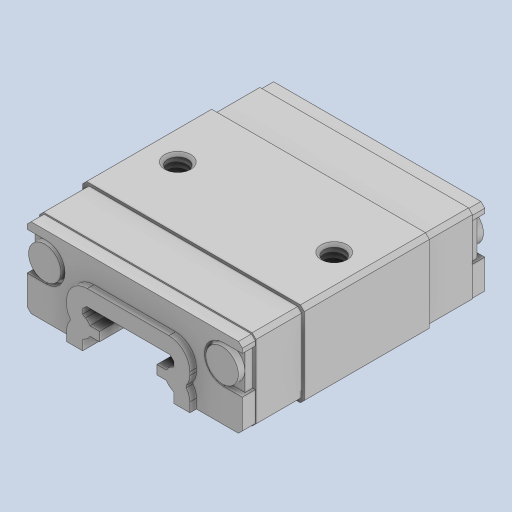
# Autodesk Inventor part: SEBSZ8_b
Saved by Autodesk Inventor 2023 (Build 270158000, 158)
## iProperties
Category: PARTsolutions
Company: MISUMI
Created: 2024-12-13
Part Number: SEBSZ8_b
Material: Generic
Catalog Web Link: www.cadenas.de
Description: SEBSZ, SE2BSZ, SSEBSZ, SSEBSZ-MX, SSE2BSZ, SSE2BSLZ-MX, SEBSLZ, SE2BSLZ, SSEBSLZ, SSEBSZ-MX, SSE2BSLZ, SSE2BSLZ-MX_block-Miniature Linear Guides - Short Block, Standard Preload
Vendor: MISUMI
Document SubType Name: Modeling
Designer: psAdmin
Manufacturer: MISUMI
Mass: 1.60852 g
Surface Area: 13.4851 cm^2
Volume: 1.60852 cm^3
Density: 1 g/cm^3
Appearance: PSOLRGB-175-175-175
PSOL_IDENT_0: {$CADENAS_DATA/23d-libs/misumi/metric/06_linear_guides/sebsz_series/sebsz_block.prj},277 {VTYP=3D},{
PSOL_IDENT_1: NB=SEBSZ8_b},{LINA=SEBSZ8},{NN=SEBSZ, SE2BSZ, SSEBSZ, SSEBSZ-MX, SSE2BSZ, SSE2BSLZ-MX, SEBSLZ, SE2BS
PSOL_IDENT_2: LZ, SSEBSLZ, SSEBSZ-MX, SSE2BSLZ, SSE2BSLZ-MX_block},{DATE=01.06.2021 05:33:07},{GEOMDATE=28.09.2020
PSOL_IDENT_3: 00:26:00},{VERSION=},{LINEID=90},{WBVAR=MAT,ST,MX},{WBNUMERIC=}  {NB=SEBSZ8_b},{LINA=SEBSZ8},{KT=DU
PSOL_IDENT_4: MMY},{PN=SEBSZ8},{TYPE=SEBSZ},{H=8},{MAT=S},{ST=S},{ST1='S', 'w/o Surface Treatment','R','Low Temper
PSOL_IDENT_5: ature Black Chrome Plating'},{MX=},{MXALG= '','w/o MX(Lubrication unit)' },{HARD=56HRC~},{STPN=},{W=
PSOL_IDENT_6: 17},{L1=19.6},{B=12},{SLL=M2x2.5},{S=2},{LL=2.5},{L2=9.6},{K=6.5},{CBB=0.3},{W1=7},{W2=5.0},{H1=4.7}
PSOL_IDENT_7: ,{CAA=0.3},{F=15},{G=5.0},{CA1=0.3},{CA2=0.3},{VA1=1.5},{HA1=1.3},{WA1=1.6677},{WA2=0.7},{RA1=1.75},
PSOL_IDENT_8: {HA2=7.4140},{POIA1=0.1140},{BHA1=13.6},{BHA2=16.5},{BHA3=16.6},{BHA5=9.7445},{BHA6=16.1},{BHA7=0.0}
PSOL_IDENT_9: ,{BHA8=0.0},{BVA1=2.40},{BVA3=0.20},{BVA4=0.30},{BVA5=6.10},{BVA6=6.20},{BCA1=0.3},{BCA2H=0.00},{BCA
PSOL_IDENT_10: 2V=0.00},{BRA1=1.45},{BRA2=1.25},{BDA1=25.00},{BHB1=9.4600},{BHB2=8.9100},{BVB1=4.3300},{BVB2=1.7485
PSOL_IDENT_11: },{BRB1=1.6},{BRB2=1.3000},{BRB3=0.0},{BHC1=3.50},{BHC2=1.0},{BHC3=0.5},{BHC4=0.4},{BHC5=0.5},{MD=5.
PSOL_IDENT_12: 5}
NB: SEBSZ8_b
NN: SEBSZ, SE2BSZ, SSEBSZ, SSEBSZ-MX, SSE2BSZ, SSE2BSLZ-MX, SEBSLZ, SE2BSLZ, SSEBSLZ, SSEBSZ-MX, SSE2BSLZ, SSE2BSLZ-MX_block
NT: Miniature Linear Guides - Short Block, Standard Preload
NBSYN: $PN._b
LINA: SEBSZ8
CATALOG: Misumi
PN: SEBSZ8
H: 8
MAT: Stainless Steel
ST: w/o Surface Treatment
MX: w/o MX(Lubrication unit)
W: 17
L1: 19.6
B: 12
SLL: M2x2.5
S: 2
LL: 2.5
L2: 9.6
K: 6.5
CBB: 0.3
W1: 7
W2: 5
H1: 4.7
CAA: 0.3
F: 15
G: 5
CA1: 0.3
CA2: 0.3
VA1: 1.5
HA1: 1.3
WA1: 1.6677
WA2: 0.7
RA1: 1.75
HA2: 7.414
POIA1: 0.114
BHA1: 13.6
BHA2: 16.5
BHA3: 16.6
BHA5: 9.7445
BHA6: 16.1
BHA7: 0
BHA8: 0
BVA1: 2.4
BVA3: 0.2
BVA4: 0.3
BVA5: 6.1
BVA6: 6.2
BCA1: 0.3
BCA2H: 0
BCA2V: 0
BRA1: 1.45
BRA2: 1.25
BDA1: 25
BHB1: 9.46
BHB2: 8.91
BVB1: 4.33
BVB2: 1.7485
BRB1: 1.6
BRB2: 1.3
BRB3: 0
BHC1: 3.5
BHC2: 1
BHC3: 0.5
BHC4: 0.4
BHC5: 0.5
MD: 5.5
SUPPLIER: MISUMI
ARTICLENO: SEBSZ8_b
BOMINFO: SEBSZ8
CREATOR: CADENAS GmbH
Title: SEBSZ8
Author: Cadenas PARTsolutions
Comments: Miniature Linear Guides - Short Block, Standard Preload
Autodesk Inventor part; units mm, degrees
ref_plane "YZ Plane" through (0, 0, 0) normal (1, 0, 0) x (0, 1, 0)
ref_plane "XZ Plane" through (0, 0, 0) normal (0, 1, 0) x (-1, 0, 0)
ref_plane "XY Plane" through (0, 0, 0) normal (0, 0, 1) x (1, 0, 0)
sketch "Sketch_1" plane through (0, 0, 0) normal (0, 0, 1) x (1, 0, 0)
  line L0 (-8.5, 1.8) -> (-8.2, 1.5)
  line L1 (-8.2, 1.5) -> (-4.8723, 1.5)
  line L2 (-4.8723, 1.5) -> (-4.6578, 1.6)
  line L3 (-4.6578, 1.6) -> (4.6578, 1.6)
  line L4 (4.6578, 1.6) -> (4.8723, 1.5)
  line L5 (4.8723, 1.5) -> (8.2, 1.5)
  line L6 (8.2, 1.5) -> (8.5, 1.8)
  line L7 (8.5, 1.8) -> (8.5, 7.7)
  line L8 (8.5, 7.7) -> (8.2, 8)
  line L9 (8.2, 8) -> (-8.2, 8)
  line L10 (-8.2, 8) -> (-8.5, 7.7)
  line L11 (-8.5, 7.7) -> (-8.5, 1.8)
  constraints: 24 end point
extrude "Extrusion1" add sketch "Sketch_1" along normal mid plane 9.6
sketch "Sketch_3" plane through (0, 0, 4.8) normal (0, 0, 1) x (1, 0, 0)
  line L0 (-8.3, 7.5) -> (-8.3, 1.9)
  line L1 (-8.3, 1.9) -> (-8, 1.6)
  line L2 (-8, 1.6) -> (8, 1.6)
  line L3 (8, 1.6) -> (8.3, 1.9)
  line L4 (8.3, 1.9) -> (8.3, 7.5)
  line L5 (8.3, 7.5) -> (8, 7.8)
  line L6 (8, 7.8) -> (-8, 7.8)
  line L7 (-8, 7.8) -> (-8.3, 7.5)
  constraints: 16 end point
extrude "Extrusion2" add sketch "Sketch_3" along normal blind 5
sketch "Sketch_4" plane through (0, 0, -4.8) normal (0, 0, 1) x (1, 0, 0)
  line L0 (-8.3, 7.5) -> (-8.3, 1.9)
  line L1 (-8.3, 1.9) -> (-8, 1.6)
  line L2 (-8, 1.6) -> (8, 1.6)
  line L3 (8, 1.6) -> (8.3, 1.9)
  line L4 (8.3, 1.9) -> (8.3, 7.5)
  line L5 (8.3, 7.5) -> (8, 7.8)
  line L6 (8, 7.8) -> (-8, 7.8)
  line L7 (-8, 7.8) -> (-8.3, 7.5)
  constraints: 16 end point
extrude "Extrusion3" add sketch "Sketch_4" against normal blind 5
sketch "Sketch_8" plane through (0, 0, 9.8) normal (0, 0, 1) x (1, 0, 0)
  line L0 (-17, 12) -> (-17, 0)
  line L1 (-17, 0) -> (17, 0)
  line L2 (17, 0) -> (17, 12)
  line L3 (17, 12) -> (-17, 12)
  line L4 (-8.25, 7.05) -> (-6.8, 7.05)
  arc A0 (-6.8, 4.15) -> (-6.8, 7.05) centre (-6.8, 5.6) ccw
  line L5 (-6.8, 4.15) -> (-8.25, 4.15)
  line L6 (-8.25, 4.15) -> (-8.25, 1.9)
  line L7 (-8.25, 1.9) -> (-7.95, 1.6)
  line L8 (-7.95, 1.6) -> (7.95, 1.6)
  line L9 (7.95, 1.6) -> (8.25, 1.9)
  line L10 (8.25, 1.9) -> (8.25, 4.15)
  line L11 (8.25, 4.15) -> (6.8, 4.15)
  arc A1 (6.8, 7.05) -> (6.8, 4.15) centre (6.8, 5.6) ccw
  line L12 (6.8, 7.05) -> (8.25, 7.05)
  line L13 (8.25, 7.05) -> (8.25, 7.4)
  line L14 (8.25, 7.4) -> (7.95, 7.7)
  line L15 (7.95, 7.7) -> (-7.95, 7.7)
  line L16 (-7.95, 7.7) -> (-8.25, 7.4)
  line L17 (-8.25, 7.4) -> (-8.25, 7.05)
  constraints: 36 end point, 4 point on circle, 2 centre point
extrude "Extrusion4" cut sketch "Sketch_8" against normal blind 1.5
sketch "Sketch_6" plane through (0, 0, 9.8) normal (0, 0, 1) x (1, 0, 0)
  line L0 (-17, 11.2) -> (-17, 1.6)
  line L1 (-17, 1.6) -> (-4.73, 1.6)
  line L2 (-4.73, 1.6) -> (-4.73, 2.3258)
  arc A0 (-4.455, 3.1254) -> (-4.73, 2.3258) centre (-3.43, 2.3257) ccw
  line L3 (-4.455, 3.1254) -> (-4.455, 3.2746)
  arc A1 (-4.73, 4.0743) -> (-4.455, 3.2746) centre (-3.43, 4.0743) ccw
  line L4 (-4.73, 4.0743) -> (-4.73, 4.33)
  arc A2 (-3.13, 5.93) -> (-4.73, 4.33) centre (-3.13, 4.33) ccw
  line L5 (-3.13, 5.93) -> (3.13, 5.93)
  arc A3 (4.73, 4.33) -> (3.13, 5.93) centre (3.13, 4.33) ccw
  line L6 (4.73, 4.33) -> (4.73, 4.0743)
  arc A4 (4.455, 3.2746) -> (4.73, 4.0743) centre (3.43, 4.0743) ccw
  line L7 (4.455, 3.2746) -> (4.455, 3.1254)
  arc A5 (4.73, 2.3258) -> (4.455, 3.1254) centre (3.43, 2.3257) ccw
  line L8 (4.73, 2.3258) -> (4.73, 1.6)
  line L9 (4.73, 1.6) -> (17, 1.6)
  line L10 (17, 1.6) -> (17, 11.2)
  line L11 (17, 11.2) -> (-17, 11.2)
  constraints: 24 end point, 12 point on circle, 6 centre point
extrude "Extrusion5" cut sketch "Sketch_6" against normal blind 0.5
sketch "Sketch_7" plane through (0, 0, -9.8) normal (0, 0, 1) x (1, 0, 0)
  line L0 (-17, 12) -> (-17, 0)
  line L1 (-17, 0) -> (17, 0)
  line L2 (17, 0) -> (17, 12)
  line L3 (17, 12) -> (-17, 12)
  line L4 (-8.25, 7.05) -> (-6.8, 7.05)
  arc A0 (-6.8, 4.15) -> (-6.8, 7.05) centre (-6.8, 5.6) ccw
  line L5 (-6.8, 4.15) -> (-8.25, 4.15)
  line L6 (-8.25, 4.15) -> (-8.25, 1.9)
  line L7 (-8.25, 1.9) -> (-7.95, 1.6)
  line L8 (-7.95, 1.6) -> (7.95, 1.6)
  line L9 (7.95, 1.6) -> (8.25, 1.9)
  line L10 (8.25, 1.9) -> (8.25, 4.15)
  line L11 (8.25, 4.15) -> (6.8, 4.15)
  arc A1 (6.8, 7.05) -> (6.8, 4.15) centre (6.8, 5.6) ccw
  line L12 (6.8, 7.05) -> (8.25, 7.05)
  line L13 (8.25, 7.05) -> (8.25, 7.4)
  line L14 (8.25, 7.4) -> (7.95, 7.7)
  line L15 (7.95, 7.7) -> (-7.95, 7.7)
  line L16 (-7.95, 7.7) -> (-8.25, 7.4)
  line L17 (-8.25, 7.4) -> (-8.25, 7.05)
  constraints: 36 end point, 4 point on circle, 2 centre point
extrude "Extrusion6" cut sketch "Sketch_7" along normal blind 1.5
sketch "Sketch_12" plane through (0, 0, -9.8) normal (0, 0, 1) x (1, 0, 0)
  line L0 (-17, 11.2) -> (-17, 1.6)
  line L1 (-17, 1.6) -> (-4.73, 1.6)
  line L2 (-4.73, 1.6) -> (-4.73, 2.3258)
  arc A0 (-4.455, 3.1254) -> (-4.73, 2.3258) centre (-3.43, 2.3257) ccw
  line L3 (-4.455, 3.1254) -> (-4.455, 3.2746)
  arc A1 (-4.73, 4.0743) -> (-4.455, 3.2746) centre (-3.43, 4.0743) ccw
  line L4 (-4.73, 4.0743) -> (-4.73, 4.33)
  arc A2 (-3.13, 5.93) -> (-4.73, 4.33) centre (-3.13, 4.33) ccw
  line L5 (-3.13, 5.93) -> (3.13, 5.93)
  arc A3 (4.73, 4.33) -> (3.13, 5.93) centre (3.13, 4.33) ccw
  line L6 (4.73, 4.33) -> (4.73, 4.0743)
  arc A4 (4.455, 3.2746) -> (4.73, 4.0743) centre (3.43, 4.0743) ccw
  line L7 (4.455, 3.2746) -> (4.455, 3.1254)
  arc A5 (4.73, 2.3258) -> (4.455, 3.1254) centre (3.43, 2.3257) ccw
  line L8 (4.73, 2.3258) -> (4.73, 1.6)
  line L9 (4.73, 1.6) -> (17, 1.6)
  line L10 (17, 1.6) -> (17, 11.2)
  line L11 (17, 11.2) -> (-17, 11.2)
  constraints: 24 end point, 12 point on circle, 6 centre point
extrude "Extrusion7" cut sketch "Sketch_12" along normal blind 0.5
sketch "Sketch_25" plane through (0, 0, 8.3) normal (0, 0, 1) x (1, 0, 0)
  line L0 (-8.05, 7.05) -> (-8.05, 4.15)
  line L1 (-8.05, 4.15) -> (-6.8, 4.15)
  arc A0 (-6.8, 4.15) -> (-6.8, 7.05) centre (-6.8, 5.6) ccw
  line L2 (-6.8, 7.05) -> (-8.05, 7.05)
  constraints: 6 end point, 2 point on circle, 1 centre point
extrude "Extrusion8" add sketch "Sketch_25" along normal blind 0.6
sketch "Sketch_5" plane through (0, 0, 8.3) normal (0, 0, 1) x (1, 0, 0)
  arc A0 (6.8, 7.05) -> (6.8, 4.15) centre (6.8, 5.6) ccw
  line L0 (6.8, 4.15) -> (8.05, 4.15)
  line L1 (8.05, 4.15) -> (8.05, 7.05)
  line L2 (8.05, 7.05) -> (6.8, 7.05)
  constraints: 6 end point, 2 point on circle, 1 centre point
extrude "Extrusion9" add sketch "Sketch_5" along normal blind 0.6
sketch "Sketch_9" plane through (0, 0, -8.3) normal (0, 0, 1) x (1, 0, 0)
  line L0 (-8.05, 7.05) -> (-8.05, 4.15)
  line L1 (-8.05, 4.15) -> (-6.8, 4.15)
  arc A0 (-6.8, 4.15) -> (-6.8, 7.05) centre (-6.8, 5.6) ccw
  line L2 (-6.8, 7.05) -> (-8.05, 7.05)
  constraints: 6 end point, 2 point on circle, 1 centre point
extrude "Extrusion10" add sketch "Sketch_9" against normal blind 0.6
sketch "Sketch_26" plane through (0, 0, -8.3) normal (0, 0, 1) x (1, 0, 0)
  arc A0 (6.8, 7.05) -> (6.8, 4.15) centre (6.8, 5.6) ccw
  line L0 (6.8, 4.15) -> (8.05, 4.15)
  line L1 (8.05, 4.15) -> (8.05, 7.05)
  line L2 (8.05, 7.05) -> (6.8, 7.05)
  constraints: 6 end point, 2 point on circle, 1 centre point
extrude "Extrusion11" add sketch "Sketch_26" against normal blind 0.6
sketch "Sketch_18" plane through (-6.8, 0, 0) normal (1, 0, 0) x (0, 0, -1)
  line L0 (-8.9, 5.6) -> (-9.4, 5.6)
  line L1 (-9.4, 5.6) -> (-9.4, 6.85)
  line L2 (-9.4, 6.85) -> (-8.9, 6.85)
  line L3 (-8.9, 6.85) -> (-8.9, 5.6)
  line L4 (-8.9, 5.6) -> (-9.4, 5.6)
  constraints: 10 end point
revolve "Revolution1" add sketch "Sketch_18" angle 360 about axis through (-6.8, 5.6, 8.9) along (0, 0, -1)
sketch "Sketch_19" plane through (-6.8, 0, 0) normal (1, 0, 0) x (0, 0, -1)
  line L0 (9.4, 5.6) -> (8.9, 5.6)
  line L1 (8.9, 5.6) -> (8.9, 6.85)
  line L2 (8.9, 6.85) -> (9.4, 6.85)
  line L3 (9.4, 6.85) -> (9.4, 5.6)
  line L4 (9.4, 5.6) -> (8.9, 5.6)
  constraints: 10 end point
revolve "Revolution2" add sketch "Sketch_19" angle 360 about axis through (-6.8, 5.6, -9.4) along (0, 0, -1)
sketch "Sketch_20" plane through (6.8, 0, 0) normal (1, 0, 0) x (0, 0, -1)
  line L0 (-8.9, 5.6) -> (-9.4, 5.6)
  line L1 (-9.4, 5.6) -> (-9.4, 6.85)
  line L2 (-9.4, 6.85) -> (-8.9, 6.85)
  line L3 (-8.9, 6.85) -> (-8.9, 5.6)
  line L4 (-8.9, 5.6) -> (-9.4, 5.6)
  constraints: 10 end point
revolve "Revolution3" add sketch "Sketch_20" angle 360 about axis through (6.8, 5.6, 8.9) along (0, 0, -1)
sketch "Sketch_21" plane through (6.8, 0, 0) normal (1, 0, 0) x (0, 0, -1)
  line L0 (9.4, 5.6) -> (8.9, 5.6)
  line L1 (8.9, 5.6) -> (8.9, 6.85)
  line L2 (8.9, 6.85) -> (9.4, 6.85)
  line L3 (9.4, 6.85) -> (9.4, 5.6)
  line L4 (9.4, 5.6) -> (8.9, 5.6)
  constraints: 10 end point
revolve "Revolution4" add sketch "Sketch_21" angle 360 about axis through (6.8, 5.6, -9.4) along (0, 0, -1)
sketch "Sketch_17" plane through (0, 0, 0) normal (0, 0, 1) x (1, 0, 0)
  line L0 (-3.5, 4.4) -> (-3.5, 4.0339)
  line L1 (-3.5, 4.0339) -> (-3.2695, 3.9008)
  arc A0 (-2.9324, 3.55) -> (-3.2695, 3.9008) centre (-3.707, 3.143) ccw
  line L2 (-2.9324, 3.55) -> (-2.2, 3.55)
  line L3 (-2.2, 3.55) -> (-2.2, 2.85)
  line L4 (-2.2, 2.85) -> (-2.9324, 2.85)
  arc A1 (-3.2695, 2.4992) -> (-2.9324, 2.85) centre (-3.707, 3.257) ccw
  line L5 (-3.2695, 2.4992) -> (-3.5, 2.3662)
  line L6 (-3.5, 2.3662) -> (-3.5, 0.3)
  line L7 (-3.5, 0.3) -> (-3.2, 0)
  line L8 (-3.2, 0) -> (3.2, 0)
  line L9 (3.2, 0) -> (3.5, 0.3)
  line L10 (3.5, 0.3) -> (3.5, 2.3662)
  line L11 (3.5, 2.3662) -> (3.2695, 2.4992)
  arc A2 (2.9324, 2.85) -> (3.2695, 2.4992) centre (3.707, 3.257) ccw
  line L12 (2.9324, 2.85) -> (2.2, 2.85)
  line L13 (2.2, 2.85) -> (2.2, 3.55)
  line L14 (2.2, 3.55) -> (2.9324, 3.55)
  arc A3 (3.2695, 3.9008) -> (2.9324, 3.55) centre (3.707, 3.143) ccw
  line L15 (3.2695, 3.9008) -> (3.5, 4.0339)
  line L16 (3.5, 4.0339) -> (3.5, 4.4)
  line L17 (3.5, 4.4) -> (3.2, 4.7)
  line L18 (3.2, 4.7) -> (-3.2, 4.7)
  line L19 (-3.2, 4.7) -> (-3.5, 4.4)
  constraints: 40 end point, 8 point on circle, 4 centre point
extrude "Extrusion12" cut sketch "Sketch_17" along normal mid plane 9.6
sketch "Sketch_11" plane through (0, 0, 4.8) normal (0, 0, 1) x (1, 0, 0)
  line L0 (-3.5, 4.4) -> (-3.5, 4.0339)
  line L1 (-3.5, 4.0339) -> (-3.2695, 3.9008)
  arc A0 (-2.9324, 3.55) -> (-3.2695, 3.9008) centre (-3.707, 3.143) ccw
  line L2 (-2.9324, 3.55) -> (-2.2, 3.55)
  line L3 (-2.2, 3.55) -> (-2.2, 2.85)
  line L4 (-2.2, 2.85) -> (-2.9324, 2.85)
  arc A1 (-3.2695, 2.4992) -> (-2.9324, 2.85) centre (-3.707, 3.257) ccw
  line L5 (-3.2695, 2.4992) -> (-3.5, 2.3662)
  line L6 (-3.5, 2.3662) -> (-3.5, 0.3)
  line L7 (-3.5, 0.3) -> (-3.2, 0)
  line L8 (-3.2, 0) -> (3.2, 0)
  line L9 (3.2, 0) -> (3.5, 0.3)
  line L10 (3.5, 0.3) -> (3.5, 2.3662)
  line L11 (3.5, 2.3662) -> (3.2695, 2.4992)
  arc A2 (2.9324, 2.85) -> (3.2695, 2.4992) centre (3.707, 3.257) ccw
  line L12 (2.9324, 2.85) -> (2.2, 2.85)
  line L13 (2.2, 2.85) -> (2.2, 3.55)
  line L14 (2.2, 3.55) -> (2.9324, 3.55)
  arc A3 (3.2695, 3.9008) -> (2.9324, 3.55) centre (3.707, 3.143) ccw
  line L15 (3.2695, 3.9008) -> (3.5, 4.0339)
  line L16 (3.5, 4.0339) -> (3.5, 4.4)
  line L17 (3.5, 4.4) -> (3.2, 4.7)
  line L18 (3.2, 4.7) -> (-3.2, 4.7)
  line L19 (-3.2, 4.7) -> (-3.5, 4.4)
  constraints: 40 end point, 8 point on circle, 4 centre point
extrude "Extrusion13" cut sketch "Sketch_11" along normal blind 9.6
sketch "Sketch_22" plane through (0, 0, 4.8) normal (0, 0, 1) x (1, 0, 0)
  line L0 (-17, 12) -> (-17, 0)
  line L1 (-17, 0) -> (17, 0)
  line L2 (17, 0) -> (17, 12)
  line L3 (17, 12) -> (-17, 12)
  line L4 (-8.3, 7.55) -> (-8.3, 2.35)
  line L5 (-8.3, 2.35) -> (-8.05, 2.1)
  line L6 (-8.05, 2.1) -> (-3.55, 2.1)
  line L7 (-3.55, 2.1) -> (-3.55, 2.4162)
  line L8 (-3.55, 2.4162) -> (-3.3467, 2.5148)
  arc A0 (-3.3467, 2.5148) -> (-2.9632, 2.9) centre (-3.707, 3.257) ccw
  line L9 (-2.9632, 2.9) -> (-2.25, 2.9)
  line L10 (-2.25, 2.9) -> (-2.25, 3.5)
  line L11 (-2.25, 3.5) -> (-2.9632, 3.5)
  arc A1 (-2.9632, 3.5) -> (-3.3467, 3.8852) centre (-3.707, 3.143) ccw
  line L12 (-3.3467, 3.8852) -> (-3.55, 3.9838)
  line L13 (-3.55, 3.9838) -> (-3.55, 4.45)
  line L14 (-3.55, 4.45) -> (-3.25, 4.75)
  line L15 (-3.25, 4.75) -> (3.25, 4.75)
  line L16 (3.25, 4.75) -> (3.55, 4.45)
  line L17 (3.55, 4.45) -> (3.55, 3.9838)
  line L18 (3.55, 3.9838) -> (3.3467, 3.8852)
  arc A2 (3.3467, 3.8852) -> (2.9632, 3.5) centre (3.707, 3.143) ccw
  line L19 (2.9632, 3.5) -> (2.25, 3.5)
  line L20 (2.25, 3.5) -> (2.25, 2.9)
  line L21 (2.25, 2.9) -> (2.9632, 2.9)
  arc A3 (2.9632, 2.9) -> (3.3467, 2.5148) centre (3.707, 3.257) ccw
  line L22 (3.3467, 2.5148) -> (3.55, 2.4162)
  line L23 (3.55, 2.4162) -> (3.55, 2.1)
  line L24 (3.55, 2.1) -> (8.05, 2.1)
  line L25 (8.05, 2.1) -> (8.3, 2.35)
  line L26 (8.3, 2.35) -> (8.3, 7.55)
  line L27 (8.3, 7.55) -> (8.05, 7.8)
  line L28 (8.05, 7.8) -> (-8.05, 7.8)
  line L29 (-8.05, 7.8) -> (-8.3, 7.55)
  constraints: 60 end point, 8 point on circle, 4 centre point
extrude "Extrusion14" cut sketch "Sketch_22" along normal blind 0.05
sketch "Sketch_10" plane through (0, 0, -4.8) normal (0, 0, 1) x (1, 0, 0)
  line L0 (-3.5, 4.4) -> (-3.5, 4.0339)
  line L1 (-3.5, 4.0339) -> (-3.2695, 3.9008)
  arc A0 (-2.9324, 3.55) -> (-3.2695, 3.9008) centre (-3.707, 3.143) ccw
  line L2 (-2.9324, 3.55) -> (-2.2, 3.55)
  line L3 (-2.2, 3.55) -> (-2.2, 2.85)
  line L4 (-2.2, 2.85) -> (-2.9324, 2.85)
  arc A1 (-3.2695, 2.4992) -> (-2.9324, 2.85) centre (-3.707, 3.257) ccw
  line L5 (-3.2695, 2.4992) -> (-3.5, 2.3662)
  line L6 (-3.5, 2.3662) -> (-3.5, 0.3)
  line L7 (-3.5, 0.3) -> (-3.2, 0)
  line L8 (-3.2, 0) -> (3.2, 0)
  line L9 (3.2, 0) -> (3.5, 0.3)
  line L10 (3.5, 0.3) -> (3.5, 2.3662)
  line L11 (3.5, 2.3662) -> (3.2695, 2.4992)
  arc A2 (2.9324, 2.85) -> (3.2695, 2.4992) centre (3.707, 3.257) ccw
  line L12 (2.9324, 2.85) -> (2.2, 2.85)
  line L13 (2.2, 2.85) -> (2.2, 3.55)
  line L14 (2.2, 3.55) -> (2.9324, 3.55)
  arc A3 (3.2695, 3.9008) -> (2.9324, 3.55) centre (3.707, 3.143) ccw
  line L15 (3.2695, 3.9008) -> (3.5, 4.0339)
  line L16 (3.5, 4.0339) -> (3.5, 4.4)
  line L17 (3.5, 4.4) -> (3.2, 4.7)
  line L18 (3.2, 4.7) -> (-3.2, 4.7)
  line L19 (-3.2, 4.7) -> (-3.5, 4.4)
  constraints: 40 end point, 8 point on circle, 4 centre point
extrude "Extrusion15" cut sketch "Sketch_10" against normal blind 9.6
sketch "Sketch_23" plane through (0, 0, -4.8) normal (0, 0, 1) x (1, 0, 0)
  line L0 (-17, 12) -> (-17, 0)
  line L1 (-17, 0) -> (17, 0)
  line L2 (17, 0) -> (17, 12)
  line L3 (17, 12) -> (-17, 12)
  line L4 (-8.3, 7.55) -> (-8.3, 2.35)
  line L5 (-8.3, 2.35) -> (-8.05, 2.1)
  line L6 (-8.05, 2.1) -> (-3.55, 2.1)
  line L7 (-3.55, 2.1) -> (-3.55, 2.4162)
  line L8 (-3.55, 2.4162) -> (-3.3467, 2.5148)
  arc A0 (-3.3467, 2.5148) -> (-2.9632, 2.9) centre (-3.707, 3.257) ccw
  line L9 (-2.9632, 2.9) -> (-2.25, 2.9)
  line L10 (-2.25, 2.9) -> (-2.25, 3.5)
  line L11 (-2.25, 3.5) -> (-2.9632, 3.5)
  arc A1 (-2.9632, 3.5) -> (-3.3467, 3.8852) centre (-3.707, 3.143) ccw
  line L12 (-3.3467, 3.8852) -> (-3.55, 3.9838)
  line L13 (-3.55, 3.9838) -> (-3.55, 4.45)
  line L14 (-3.55, 4.45) -> (-3.25, 4.75)
  line L15 (-3.25, 4.75) -> (3.25, 4.75)
  line L16 (3.25, 4.75) -> (3.55, 4.45)
  line L17 (3.55, 4.45) -> (3.55, 3.9838)
  line L18 (3.55, 3.9838) -> (3.3467, 3.8852)
  arc A2 (3.3467, 3.8852) -> (2.9632, 3.5) centre (3.707, 3.143) ccw
  line L19 (2.9632, 3.5) -> (2.25, 3.5)
  line L20 (2.25, 3.5) -> (2.25, 2.9)
  line L21 (2.25, 2.9) -> (2.9632, 2.9)
  arc A3 (2.9632, 2.9) -> (3.3467, 2.5148) centre (3.707, 3.257) ccw
  line L22 (3.3467, 2.5148) -> (3.55, 2.4162)
  line L23 (3.55, 2.4162) -> (3.55, 2.1)
  line L24 (3.55, 2.1) -> (8.05, 2.1)
  line L25 (8.05, 2.1) -> (8.3, 2.35)
  line L26 (8.3, 2.35) -> (8.3, 7.55)
  line L27 (8.3, 7.55) -> (8.05, 7.8)
  line L28 (8.05, 7.8) -> (-8.05, 7.8)
  line L29 (-8.05, 7.8) -> (-8.3, 7.55)
  constraints: 60 end point, 8 point on circle, 4 centre point
extrude "Extrusion16" cut sketch "Sketch_23" against normal blind 0.05
sketch "Sketch21" plane through (-8.2, 8, 4.8) normal (0, 1, 0) x (1, 0, 0)
  point P0 (2.2, 4.8)
hole "Hole1" at (-6, 8, 0) direction (0, -1, 0) diameter 1.567 depth 5.5 tip angle 120 countersink diameter 2 countersink angle 90 thread size "M2x0.4" class "6H" standard "ISO Metric profile"
pattern_linear "Rectangular Pattern1" count 2 spacing 12 along (1, 0, 0) of "Hole1"
ref_plane "to_rail_XY" through (0, 4.7, 0) normal (0, 0, -1) x (1, 0, 0)
ref_plane "to_rail_YZ" through (0, 4.7, 0) normal (1, 0, 0) x (0, -1, 0)
ref_plane "to_rail_ZX" through (0, 4.7, 0) normal (0, -1, 0) x (0, 0, -1)
body "Solid1"
